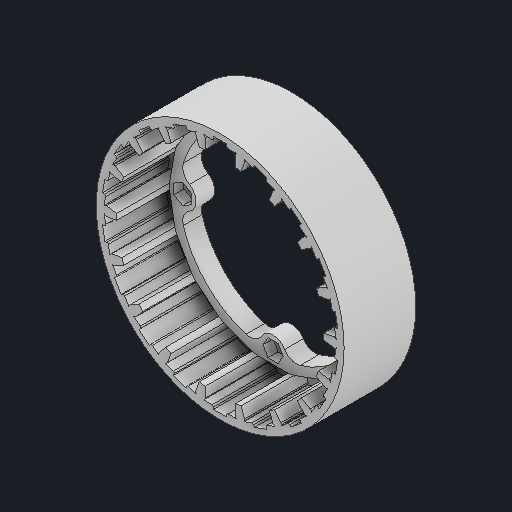
# Autodesk Inventor part: Rotator_A
Saved by Autodesk Inventor 2025.1 (Build 291241020, 241B)
## iProperties
Created: 2025-07-24
Part Number: Rotator_A
Material: 일반
Document SubType Name: Modeling
Designer: acalo
Density: 1 g/cm^3
Appearance: 기본값
Author: acalo
Autodesk Inventor part; units mm, degrees
ref_plane "YZ Plane" through (0, 0, 0) normal (1, 0, 0) x (0, 1, 0)
ref_plane "XZ Plane" through (0, 0, 0) normal (0, 1, 0) x (-1, 0, 0)
ref_plane "XY Plane" through (0, 0, 0) normal (0, 0, 1) x (1, 0, 0)
sketch "스케치1" plane through (0, 0, 0) normal (0, 0, 1) x (1, 0, 0)
  circle A0 centre (0, 0) radius 30
  line L0 (0, 30) -> (0, 30.6)
  line L1 (0, 30.6) -> (4.5, 30.6)
  line L2 (4.5, 30.6) -> (4.5, 34.2)
  line L3 (4.5, 34.2) -> (-4.5, 34.2)
  line L4 (-4.5, 34.2) -> (-4.5, 30.6)
  line L5 (-4.5, 30.6) -> (0, 30.6)
  line L6 (-10.4658, 28.7546) -> (-6.2372, 30.2937)
  line L7 (-6.2372, 30.2937) -> (-7.4685, 33.6766)
  line L8 (-7.4685, 33.6766) -> (-15.9257, 30.5984)
  line L9 (-15.9257, 30.5984) -> (-14.6944, 27.2155)
  line L10 (-14.6944, 27.2155) -> (-10.4658, 28.7546)
  line L11 (-19.6693, 23.441) -> (-16.2221, 26.3335)
  line L12 (-16.2221, 26.3335) -> (-18.5361, 29.0913)
  line L13 (-18.5361, 29.0913) -> (-25.4305, 23.3062)
  line L14 (-25.4305, 23.3062) -> (-23.1165, 20.5484)
  line L15 (-23.1165, 20.5484) -> (-19.6693, 23.441)
  line L16 (-26.5004, 15.3) -> (-24.2504, 19.1971)
  line L17 (-24.2504, 19.1971) -> (-27.3681, 20.9971)
  line L18 (-27.3681, 20.9971) -> (-31.8681, 13.2029)
  line L19 (-31.8681, 13.2029) -> (-28.7504, 11.4029)
  line L20 (-28.7504, 11.4029) -> (-26.5004, 15.3)
  line L21 (-30.1351, 5.3136) -> (-29.3537, 9.7453)
  line L22 (-29.3537, 9.7453) -> (-32.899, 10.3704)
  line L23 (-32.899, 10.3704) -> (-34.4618, 1.5071)
  line L24 (-34.4618, 1.5071) -> (-30.9165, 0.882)
  line L25 (-30.9165, 0.882) -> (-30.1351, 5.3136)
  line L26 (-30.1351, -5.3136) -> (-30.9165, -0.882)
  line L27 (-30.9165, -0.882) -> (-34.4618, -1.5071)
  line L28 (-34.4618, -1.5071) -> (-32.899, -10.3704)
  line L29 (-32.899, -10.3704) -> (-29.3537, -9.7453)
  line L30 (-29.3537, -9.7453) -> (-30.1351, -5.3136)
  line L31 (-26.5004, -15.3) -> (-28.7504, -11.4029)
  line L32 (-28.7504, -11.4029) -> (-31.8681, -13.2029)
  line L33 (-31.8681, -13.2029) -> (-27.3681, -20.9971)
  line L34 (-27.3681, -20.9971) -> (-24.2504, -19.1971)
  line L35 (-24.2504, -19.1971) -> (-26.5004, -15.3)
  line L36 (-19.6693, -23.441) -> (-23.1165, -20.5484)
  line L37 (-23.1165, -20.5484) -> (-25.4305, -23.3062)
  line L38 (-25.4305, -23.3062) -> (-18.5361, -29.0913)
  line L39 (-18.5361, -29.0913) -> (-16.2221, -26.3335)
  line L40 (-16.2221, -26.3335) -> (-19.6693, -23.441)
  line L41 (-10.4658, -28.7546) -> (-14.6944, -27.2155)
  line L42 (-14.6944, -27.2155) -> (-15.9257, -30.5984)
  line L43 (-15.9257, -30.5984) -> (-7.4685, -33.6766)
  line L44 (-7.4685, -33.6766) -> (-6.2372, -30.2937)
  line L45 (-6.2372, -30.2937) -> (-10.4658, -28.7546)
  line L46 (0, -30.6) -> (-4.5, -30.6)
  line L47 (-4.5, -30.6) -> (-4.5, -34.2)
  line L48 (-4.5, -34.2) -> (4.5, -34.2)
  line L49 (4.5, -34.2) -> (4.5, -30.6)
  line L50 (4.5, -30.6) -> (0, -30.6)
  line L51 (10.4658, -28.7546) -> (6.2372, -30.2937)
  line L52 (6.2372, -30.2937) -> (7.4685, -33.6766)
  line L53 (7.4685, -33.6766) -> (15.9257, -30.5984)
  line L54 (15.9257, -30.5984) -> (14.6944, -27.2155)
  line L55 (14.6944, -27.2155) -> (10.4658, -28.7546)
  line L56 (19.6693, -23.441) -> (16.2221, -26.3335)
  line L57 (16.2221, -26.3335) -> (18.5361, -29.0913)
  line L58 (18.5361, -29.0913) -> (25.4305, -23.3062)
  line L59 (25.4305, -23.3062) -> (23.1165, -20.5484)
  line L60 (23.1165, -20.5484) -> (19.6693, -23.441)
  line L61 (26.5004, -15.3) -> (24.2504, -19.1971)
  line L62 (24.2504, -19.1971) -> (27.3681, -20.9971)
  line L63 (27.3681, -20.9971) -> (31.8681, -13.2029)
  line L64 (31.8681, -13.2029) -> (28.7504, -11.4029)
  line L65 (28.7504, -11.4029) -> (26.5004, -15.3)
  line L66 (30.1351, -5.3136) -> (29.3537, -9.7453)
  line L67 (29.3537, -9.7453) -> (32.899, -10.3704)
  line L68 (32.899, -10.3704) -> (34.4618, -1.5071)
  line L69 (34.4618, -1.5071) -> (30.9165, -0.882)
  line L70 (30.9165, -0.882) -> (30.1351, -5.3136)
  line L71 (30.1351, 5.3136) -> (30.9165, 0.882)
  line L72 (30.9165, 0.882) -> (34.4618, 1.5071)
  line L73 (34.4618, 1.5071) -> (32.899, 10.3704)
  line L74 (32.899, 10.3704) -> (29.3537, 9.7453)
  line L75 (29.3537, 9.7453) -> (30.1351, 5.3136)
  line L76 (26.5004, 15.3) -> (28.7504, 11.4029)
  line L77 (28.7504, 11.4029) -> (31.8681, 13.2029)
  line L78 (31.8681, 13.2029) -> (27.3681, 20.9971)
  line L79 (27.3681, 20.9971) -> (24.2504, 19.1971)
  line L80 (24.2504, 19.1971) -> (26.5004, 15.3)
  line L81 (19.6693, 23.441) -> (23.1165, 20.5484)
  line L82 (23.1165, 20.5484) -> (25.4305, 23.3062)
  line L83 (25.4305, 23.3062) -> (18.5361, 29.0913)
  line L84 (18.5361, 29.0913) -> (16.2221, 26.3335)
  line L85 (16.2221, 26.3335) -> (19.6693, 23.441)
  line L86 (10.4658, 28.7546) -> (14.6944, 27.2155)
  line L87 (14.6944, 27.2155) -> (15.9257, 30.5984)
  line L88 (15.9257, 30.5984) -> (7.4685, 33.6766)
  line L89 (7.4685, 33.6766) -> (6.2372, 30.2937)
  line L90 (6.2372, 30.2937) -> (10.4658, 28.7546)
  circle A1 centre (0, 0) radius 28
  circle A2 centre (0, 0) radius 37
  line L91 (-4.5, 30.6) -> (-6.2372, 30.2937)
  line L92 (-14.6944, 27.2155) -> (-16.2221, 26.3335)
  line L93 (-23.1165, 20.5484) -> (-24.2504, 19.1971)
  line L94 (-28.7504, 11.4029) -> (-29.3537, 9.7453)
  line L95 (-30.9165, 0.882) -> (-30.9165, -0.882)
  line L96 (-29.3537, -9.7453) -> (-28.7504, -11.4029)
  line L97 (-24.2504, -19.1971) -> (-23.1165, -20.5484)
  line L98 (-16.2221, -26.3335) -> (-14.6944, -27.2155)
  line L99 (-6.2372, -30.2937) -> (-4.5, -30.6)
  line L100 (4.5, -30.6) -> (6.2372, -30.2937)
  line L101 (14.6944, -27.2155) -> (16.2221, -26.3335)
  line L102 (23.1165, -20.5484) -> (24.2504, -19.1971)
  line L103 (28.7504, -11.4029) -> (29.3537, -9.7453)
  line L104 (30.9165, -0.882) -> (30.9165, 0.882)
  line L105 (29.3537, 9.7453) -> (28.7504, 11.4029)
  line L106 (24.2504, 19.1971) -> (23.1165, 20.5484)
  line L107 (16.2221, 26.3335) -> (14.6944, 27.2155)
  line L108 (6.2372, 30.2937) -> (4.5, 30.6)
  dimension "d1" = 0.6
  dimension "d2" = 4.5
  dimension "d3" = 3.6
  dimension "d4" = 9
  dimension "d7" = 360
  dimension "d9" = 56
  dimension "d10" = 74
  dimension "d13" = 360
  constraints: 218 end point, 18 point on line, 4 perpendicular, 3 coincident, 2 centre point, 1 horizontal, 1 vertical, 1 vertical alignment, 238 other
  measures "d1" distance of L0.start L0.end
  measures "d2" distance of L0.end L1.end
  measures "d3" distance of L1.end L2.end
  measures "d4" distance of L2.end L3.end
  measures "d9" diameter of A1
  measures "d10" diameter of A2
extrude "돌출1" add sketch "스케치1" along normal blind 19 contours A2
extrude "돌출2" add sketch "스케치1" against normal blind 2.4 contours A0 | L5 L4 L3 L2 L1 | L1 L108 L90 L86 L107 L85 L81 L106 L80 L76 L105 L75 L71 L104 L70 L66 L103 L65 L61 L102 L60 L56 L101 L55 L51 L100 L50 L46 L99 L45 L41 L98 L40 L36 L97 L35 L31 L96 L30 L26 L95 L25 L21 L94 L20 L16 L93 L15 L11 L92 L10 L6 L91 L5 | L89 L88 L87 L86 L90 | L6 L10 L9 L8 L7 | L84 L83 L82 L81 L85 | L11 L15 L14 L13 L12 | L79 L78 L77 L76 L80 | L16 L20 L19 L18 L17 | L74 L73 L72 L71 L75 | L21 L25 L24 L23 L22 | L69 L68 L67 L66 L70 | L26 L30 L29 L28 L27 | L64 L63 L62 L61 L65 | L31 L35 L34 L33 L32 | L59 L58 L57 L56 L60 | L36 L40 L39 L38 L37 | L54 L53 L52 L51 L55 | L41 L45 L44 L43 L42 | L49 L48 L47 L46 L50 | A2
extrude "돌출3" add sketch "스케치1" along normal blind 2 contours A0 | L1 L108 L90 L86 L107 L85 L81 L106 L80 L76 L105 L75 L71 L104 L70 L66 L103 L65 L61 L102 L60 L56 L101 L55 L51 L100 L50 L46 L99 L45 L41 L98 L40 L36 L97 L35 L31 L96 L30 L26 L95 L25 L21 L94 L20 L16 L93 L15 L11 L92 L10 L6 L91 L5
sketch "스케치2" plane through (0, 0, 19) normal (0, 0, 1) x (1, 0, 0)
  circle A0 centre (0, 0) radius 37 projected
  line L0 (4.5, 30.6) -> (6.2372, 30.2937) projected
  line L1 (6.2372, 30.2937) -> (7.4685, 33.6766) projected
  line L2 (7.4685, 33.6766) -> (15.9257, 30.5984) projected
  line L3 (15.9257, 30.5984) -> (14.6944, 27.2155) projected
  line L4 (14.6944, 27.2155) -> (16.2221, 26.3335) projected
  line L5 (16.2221, 26.3335) -> (18.5361, 29.0913) projected
  line L6 (18.5361, 29.0913) -> (25.4305, 23.3062) projected
  line L7 (25.4305, 23.3062) -> (23.1165, 20.5484) projected
  line L8 (23.1165, 20.5484) -> (24.2504, 19.1971) projected
  line L9 (24.2504, 19.1971) -> (27.3681, 20.9971) projected
  line L10 (27.3681, 20.9971) -> (31.8681, 13.2029) projected
  line L11 (31.8681, 13.2029) -> (28.7504, 11.4029) projected
  line L12 (28.7504, 11.4029) -> (29.3537, 9.7453) projected
  line L13 (29.3537, 9.7453) -> (32.899, 10.3704) projected
  line L14 (32.899, 10.3704) -> (34.4618, 1.5071) projected
  line L15 (34.4618, 1.5071) -> (30.9165, 0.882) projected
  line L16 (30.9165, 0.882) -> (30.9165, -0.882) projected
  line L17 (30.9165, -0.882) -> (34.4618, -1.5071) projected
  line L18 (34.4618, -1.5071) -> (32.899, -10.3704) projected
  line L19 (32.899, -10.3704) -> (29.3537, -9.7453) projected
  line L20 (29.3537, -9.7453) -> (28.7504, -11.4029) projected
  line L21 (28.7504, -11.4029) -> (31.8681, -13.2029) projected
  line L22 (31.8681, -13.2029) -> (27.3681, -20.9971) projected
  line L23 (27.3681, -20.9971) -> (24.2504, -19.1971) projected
  line L24 (24.2504, -19.1971) -> (23.1165, -20.5484) projected
  line L25 (23.1165, -20.5484) -> (25.4305, -23.3062) projected
  line L26 (25.4305, -23.3062) -> (18.5361, -29.0913) projected
  line L27 (18.5361, -29.0913) -> (16.2221, -26.3335) projected
  line L28 (16.2221, -26.3335) -> (14.6944, -27.2155) projected
  line L29 (14.6944, -27.2155) -> (15.9257, -30.5984) projected
  line L30 (15.9257, -30.5984) -> (7.4685, -33.6766) projected
  line L31 (7.4685, -33.6766) -> (6.2372, -30.2937) projected
  line L32 (6.2372, -30.2937) -> (4.5, -30.6) projected
  line L33 (4.5, -30.6) -> (4.5, -34.2) projected
  line L34 (4.5, -34.2) -> (-4.5, -34.2) projected
  line L35 (-4.5, -34.2) -> (-4.5, -30.6) projected
  line L36 (-4.5, -30.6) -> (-6.2372, -30.2937) projected
  line L37 (-6.2372, -30.2937) -> (-7.4685, -33.6766) projected
  line L38 (-7.4685, -33.6766) -> (-15.9257, -30.5984) projected
  line L39 (-15.9257, -30.5984) -> (-14.6944, -27.2155) projected
  line L40 (-14.6944, -27.2155) -> (-16.2221, -26.3335) projected
  line L41 (-16.2221, -26.3335) -> (-18.5361, -29.0913) projected
  line L42 (-18.5361, -29.0913) -> (-25.4305, -23.3062) projected
  line L43 (-25.4305, -23.3062) -> (-23.1165, -20.5484) projected
  line L44 (-23.1165, -20.5484) -> (-24.2504, -19.1971) projected
  line L45 (-24.2504, -19.1971) -> (-27.3681, -20.9971) projected
  line L46 (-27.3681, -20.9971) -> (-31.8681, -13.2029) projected
  line L47 (-31.8681, -13.2029) -> (-28.7504, -11.4029) projected
  line L48 (-28.7504, -11.4029) -> (-29.3537, -9.7453) projected
  line L49 (-29.3537, -9.7453) -> (-32.899, -10.3704) projected
  line L50 (-32.899, -10.3704) -> (-34.4618, -1.5071) projected
  line L51 (-34.4618, -1.5071) -> (-30.9165, -0.882) projected
  line L52 (-30.9165, -0.882) -> (-30.9165, 0.882) projected
  line L53 (-30.9165, 0.882) -> (-34.4618, 1.5071) projected
  line L54 (-34.4618, 1.5071) -> (-32.899, 10.3704) projected
  line L55 (-32.899, 10.3704) -> (-29.3537, 9.7453) projected
  line L56 (-29.3537, 9.7453) -> (-28.7504, 11.4029) projected
  line L57 (-28.7504, 11.4029) -> (-31.8681, 13.2029) projected
  line L58 (-31.8681, 13.2029) -> (-27.3681, 20.9971) projected
  line L59 (-27.3681, 20.9971) -> (-24.2504, 19.1971) projected
  line L60 (-24.2504, 19.1971) -> (-23.1165, 20.5484) projected
  line L61 (-23.1165, 20.5484) -> (-25.4305, 23.3062) projected
  line L62 (-25.4305, 23.3062) -> (-18.5361, 29.0913) projected
  line L63 (-18.5361, 29.0913) -> (-16.2221, 26.3335) projected
  line L64 (-16.2221, 26.3335) -> (-14.6944, 27.2155) projected
  line L65 (-14.6944, 27.2155) -> (-15.9257, 30.5984) projected
  line L66 (-15.9257, 30.5984) -> (-7.4685, 33.6766) projected
  line L67 (-7.4685, 33.6766) -> (-6.2372, 30.2937) projected
  line L68 (-6.2372, 30.2937) -> (-4.5, 30.6) projected
  line L69 (-4.5, 30.6) -> (-4.5, 34.2) projected
  line L70 (-4.5, 34.2) -> (4.5, 34.2) projected
  line L71 (4.5, 34.2) -> (4.5, 30.6) projected
  line L72 (37, 0) -> (38.2, 0)
  circle A1 centre (38.2, 0) radius 1.65
  line L73 (38.2, 0) -> (42.2, 0)
  arc A2 (42.01, -4) -> (42.01, 4) centre (0, 0) ccw
  line L74 (36.7831, 4) -> (42.01, 4)
  line L75 (36.7831, -4) -> (42.01, -4)
  point P0 (38.2, 4)
  point P1 (40.3945, 4)
  point P2 (38.2, -4)
  point P3 (40.3945, -4)
  point P4 (36.9832, 1.1144)
  point P5 (36.9832, -1.1144)
  dimension "d22" = 3.3
  dimension "d27" = 4
  constraints: 8 end point, 6 point on circle, 4 point on line, 2 centre point, 2 coincident, 2 horizontal, 2 symmetric about line
  measures "d22" diameter of A1
  measures "d27" distance of L73.start L73.end
thicken "두껍게 하기1" operation add thickness 1.2 both sides no extend neighbours no toward (0, 0, 1) faces at (-1.125, 29.6653, 2)
sketch "스케치3" plane through (0, 0, 19) normal (0, 0, 1) x (1, 0, 0)
  line L0 (4.2, -34.2) -> (-4.2, -34.2)
  line L1 (4.5, -34.2) -> (-4.5, -34.2)
  line L2 (0, -35.2) -> (-2, -35.2)
  line L3 (-2, -35.2) -> (-2, -34.2)
  line L4 (0, -35.2) -> (2, -35.2)
  line L5 (2, -35.2) -> (2, -34.2)
  point P0 (0, 0)
  dimension "d40" = 2
  constraints: 12 end point, 2 point on line
  measures "d40" distance of L2.start L2.end
extrude "돌출6" cut sketch "스케치3" against normal up to surface (19 mm away)
fillet "모깎기3" radius 0.4 2 edges at (2, -34.2, 9.5) (-2, -34.2, 9.5)
pattern_circular "원형 패턴3" count 18 over 360 about axis through (0, 0, 0) along (0, 0, -1) of "모깎기3", "돌출6"
ref_plane "작업 평면1" through (-4.2, -30.6, 3.2) normal (0, 0, 1) x (1, 0, 0)
sketch "스케치4" plane through (-4.2, -30.6, 3.2) normal (0, 0, 1) x (1, 0, 0)
  circle A0 centre (4.2, 30.6) radius 28 projected
  circle A1 centre (31.2, 30.6) radius 1.65
  line L0 (31.2, 34.6) -> (33.9128, 34.6)
  line L1 (31.2, 26.6) -> (33.9128, 26.6)
  arc A2 (31.2, 34.6) -> (31.2, 26.6) centre (31.2, 30.6) ccw
  line L2 (9.911, 34.0794) -> (11.911, 34.0794)
  point P0 (30.85, 34.6)
  point P1 (30.85, 26.6)
  point P2 (31.9128, 34.6)
  point P3 (31.9128, 26.6)
  point P4 (32.1681, 29.2639)
  point P5 (32.1681, 31.9361)
  dimension "d49" = 3.3
  dimension "d59" = 2
  constraints: 6 end point, 2 centre point, 2 horizontal, 2 point on circle, 1 coincident, 1 tangent
  measures "d49" diameter of A1
  measures "d59" distance of L2.start L2.end
extrude "돌출10" add sketch "스케치4" against normal up to surface (5.6 mm away) contours A1 A0 L1 A2 L0
extrude "돌출11" cut sketch "스케치4" against normal up to surface (5.6 mm away) contours A0 A1 | L0 A2 L1 A0 picked at (32.4002, 30.3229)
ref_plane "작업 평면2" through (-4.2, -30.6, 3.2) normal (0, 0, 1) x (1, 0, 0)
sketch "스케치7" plane through (-4.2, -30.6, 3.2) normal (0, 0, 1) x (1, 0, 0)
  circle A0 centre (31.2, 30.6) radius 1.65
  arc A1 (31.0117, 38.6704) -> (31.0117, 22.5296) centre (4.2, 30.6) ccw
  arc A2 (29.1907, 34.0587) -> (31.0117, 38.6704) centre (27.1815, 37.5175) ccw
  arc A3 (29.1907, 34.0587) -> (29.1907, 27.1413) centre (31.2, 30.6) ccw
  arc A4 (31.0117, 22.5296) -> (29.1907, 27.1413) centre (27.1815, 23.6825) ccw
  line L0 (-2.0372, 60.8937) -> (-0.3, 61.2) projected
  line L1 (-2.1398, 61.1756) -> (-2.0372, 60.8937) projected
  arc A5 (-2.3191, 60.7911) -> (-2.1398, 61.1756) centre (-2.4217, 61.073) ccw projected
  line L2 (-2.3191, 60.7911) -> (-10.2125, 57.9181) projected
  arc A6 (-10.597, 58.0974) -> (-10.2125, 57.9181) centre (-10.3151, 58.2) ccw projected
  line L3 (-10.4944, 57.8155) -> (-10.597, 58.0974) projected
  line L4 (-12.0221, 56.9335) -> (-10.4944, 57.8155) projected
  line L5 (-12.2149, 57.1633) -> (-12.0221, 56.9335) projected
  arc A7 (-12.2519, 56.7407) -> (-12.2149, 57.1633) centre (-12.4448, 56.9705) ccw projected
  line L6 (-12.2519, 56.7407) -> (-18.6867, 51.3413) projected
  arc A8 (-19.1093, 51.3782) -> (-18.6867, 51.3413) centre (-18.8795, 51.5711) ccw projected
  line L7 (-18.9165, 51.1484) -> (-19.1093, 51.3782) projected
  line L8 (-20.0504, 49.7971) -> (-18.9165, 51.1484) projected
  line L9 (-20.3102, 49.9471) -> (-20.0504, 49.7971) projected
  arc A9 (-20.2004, 49.5373) -> (-20.3102, 49.9471) centre (-20.4602, 49.6873) ccw projected
  line L10 (-20.2004, 49.5373) -> (-24.4004, 42.2627) projected
  arc A10 (-24.8102, 42.1529) -> (-24.4004, 42.2627) centre (-24.6602, 42.4127) ccw projected
  line L11 (-24.5504, 42.0029) -> (-24.8102, 42.1529) projected
  line L12 (-25.1537, 40.3453) -> (-24.5504, 42.0029) projected
  line L13 (-25.4491, 40.3974) -> (-25.1537, 40.3453) projected
  arc A11 (-25.2058, 40.0498) -> (-25.4491, 40.3974) centre (-25.5012, 40.1019) ccw projected
  line L14 (-25.2058, 40.0498) -> (-26.6644, 31.7774) projected
  arc A12 (-27.012, 31.5341) -> (-26.6644, 31.7774) centre (-26.9599, 31.8295) ccw projected
  line L15 (-26.7165, 31.482) -> (-27.012, 31.5341) projected
  line L16 (-26.7165, 29.718) -> (-26.7165, 31.482) projected
  line L17 (-27.012, 29.6659) -> (-26.7165, 29.718) projected
  arc A13 (-26.6644, 29.4226) -> (-27.012, 29.6659) centre (-26.9599, 29.3705) ccw projected
  line L18 (-26.6644, 29.4226) -> (-25.2058, 21.1502) projected
  arc A14 (-25.4491, 20.8026) -> (-25.2058, 21.1502) centre (-25.5012, 21.0981) ccw projected
  line L19 (-25.1537, 20.8547) -> (-25.4491, 20.8026) projected
  line L20 (-24.5504, 19.1971) -> (-25.1537, 20.8547) projected
  line L21 (-24.8102, 19.0471) -> (-24.5504, 19.1971) projected
  arc A15 (-24.4004, 18.9373) -> (-24.8102, 19.0471) centre (-24.6602, 18.7873) ccw projected
  line L22 (-24.4004, 18.9373) -> (-20.2004, 11.6627) projected
  arc A16 (-20.3102, 11.2529) -> (-20.2004, 11.6627) centre (-20.4602, 11.5127) ccw projected
  line L23 (-20.0504, 11.4029) -> (-20.3102, 11.2529) projected
  line L24 (-18.9165, 10.0516) -> (-20.0504, 11.4029) projected
  line L25 (-19.1093, 9.8218) -> (-18.9165, 10.0516) projected
  arc A17 (-18.6867, 9.8587) -> (-19.1093, 9.8218) centre (-18.8795, 9.6289) ccw projected
  line L26 (-18.6867, 9.8587) -> (-12.2519, 4.4593) projected
  arc A18 (-12.2149, 4.0367) -> (-12.2519, 4.4593) centre (-12.4448, 4.2295) ccw projected
  line L27 (-12.0221, 4.2665) -> (-12.2149, 4.0367) projected
  line L28 (-10.4944, 3.3845) -> (-12.0221, 4.2665) projected
  line L29 (-10.597, 3.1026) -> (-10.4944, 3.3845) projected
  arc A19 (-10.2125, 3.2819) -> (-10.597, 3.1026) centre (-10.3151, 3) ccw projected
  line L30 (-10.2125, 3.2819) -> (-2.3191, 0.4089) projected
  arc A20 (-2.1398, 0.0244) -> (-2.3191, 0.4089) centre (-2.4217, 0.127) ccw projected
  line L31 (-2.0372, 0.3063) -> (-2.1398, 0.0244) projected
  line L32 (-0.3, 0) -> (-2.0372, 0.3063) projected
  line L33 (-0.3, -0.3) -> (-0.3, 0) projected
  arc A21 (0, 0) -> (-0.3, -0.3) centre (0, -0.3) ccw projected
  line L34 (0, 0) -> (8.4, 0) projected
  arc A22 (8.7, -0.3) -> (8.4, 0) centre (8.4, -0.3) ccw projected
  line L35 (8.7, 0) -> (8.7, -0.3) projected
  line L36 (10.4372, 0.3063) -> (8.7, 0) projected
  line L37 (10.5398, 0.0244) -> (10.4372, 0.3063) projected
  arc A23 (10.7191, 0.4089) -> (10.5398, 0.0244) centre (10.8217, 0.127) ccw projected
  line L38 (10.7191, 0.4089) -> (18.6125, 3.2819) projected
  arc A24 (18.997, 3.1026) -> (18.6125, 3.2819) centre (18.7151, 3) ccw projected
  line L39 (18.8944, 3.3845) -> (18.997, 3.1026) projected
  line L40 (20.4221, 4.2665) -> (18.8944, 3.3845) projected
  line L41 (20.6149, 4.0367) -> (20.4221, 4.2665) projected
  arc A25 (20.6519, 4.4593) -> (20.6149, 4.0367) centre (20.8448, 4.2295) ccw projected
  line L42 (20.6519, 4.4593) -> (27.0867, 9.8587) projected
  arc A26 (27.5093, 9.8218) -> (27.0867, 9.8587) centre (27.2795, 9.6289) ccw projected
  line L43 (27.3165, 10.0516) -> (27.5093, 9.8218) projected
  line L44 (28.4504, 11.4029) -> (27.3165, 10.0516) projected
  line L45 (28.7102, 11.2529) -> (28.4504, 11.4029) projected
  arc A27 (28.6004, 11.6627) -> (28.7102, 11.2529) centre (28.8602, 11.5127) ccw projected
  line L46 (28.6004, 11.6627) -> (32.8004, 18.9373)
  arc A28 (33.2102, 19.0471) -> (32.8004, 18.9373) centre (33.0602, 18.7873) ccw
  line L47 (32.9504, 19.1971) -> (33.2102, 19.0471)
  line L48 (33.5537, 20.8547) -> (32.9504, 19.1971)
  line L49 (33.8491, 20.8026) -> (33.5537, 20.8547)
  arc A29 (33.6058, 21.1502) -> (33.8491, 20.8026) centre (33.9012, 21.0981) ccw
  line L50 (33.6058, 21.1502) -> (35.0644, 29.4226)
  arc A30 (35.412, 29.6659) -> (35.0644, 29.4226) centre (35.3599, 29.3705) ccw
  line L51 (35.1165, 29.718) -> (35.412, 29.6659)
  line L52 (35.1165, 31.482) -> (35.1165, 29.718)
  line L53 (35.412, 31.5341) -> (35.1165, 31.482)
  arc A31 (35.0644, 31.7774) -> (35.412, 31.5341) centre (35.3599, 31.8295) ccw
  line L54 (35.0644, 31.7774) -> (33.6058, 40.0498)
  arc A32 (33.8491, 40.3974) -> (33.6058, 40.0498) centre (33.9012, 40.1019) ccw
  line L55 (33.5537, 40.3453) -> (33.8491, 40.3974)
  line L56 (32.9504, 42.0029) -> (33.5537, 40.3453)
  line L57 (33.2102, 42.1529) -> (32.9504, 42.0029)
  arc A33 (32.8004, 42.2627) -> (33.2102, 42.1529) centre (33.0602, 42.4127) ccw
  line L58 (32.8004, 42.2627) -> (28.6004, 49.5373)
  arc A34 (28.7102, 49.9471) -> (28.6004, 49.5373) centre (28.8602, 49.6873) ccw projected
  line L59 (28.4504, 49.7971) -> (28.7102, 49.9471) projected
  line L60 (27.3165, 51.1484) -> (28.4504, 49.7971) projected
  line L61 (27.5093, 51.3782) -> (27.3165, 51.1484) projected
  arc A35 (27.0867, 51.3413) -> (27.5093, 51.3782) centre (27.2795, 51.5711) ccw projected
  line L62 (27.0867, 51.3413) -> (20.6519, 56.7407) projected
  arc A36 (20.6149, 57.1633) -> (20.6519, 56.7407) centre (20.8448, 56.9705) ccw projected
  line L63 (20.4221, 56.9335) -> (20.6149, 57.1633) projected
  line L64 (18.8944, 57.8155) -> (20.4221, 56.9335) projected
  line L65 (18.997, 58.0974) -> (18.8944, 57.8155) projected
  arc A37 (18.6125, 57.9181) -> (18.997, 58.0974) centre (18.7151, 58.2) ccw projected
  line L66 (18.6125, 57.9181) -> (10.7191, 60.7911) projected
  arc A38 (10.5398, 61.1756) -> (10.7191, 60.7911) centre (10.8217, 61.073) ccw projected
  line L67 (10.4372, 60.8937) -> (10.5398, 61.1756) projected
  line L68 (8.7, 61.2) -> (10.4372, 60.8937) projected
  line L69 (8.7, 61.5) -> (8.7, 61.2) projected
  arc A39 (8.4, 61.2) -> (8.7, 61.5) centre (8.4, 61.5) ccw projected
  line L70 (8.4, 61.2) -> (0, 61.2) projected
  arc A40 (-0.3, 61.5) -> (0, 61.2) centre (0, 61.5) ccw projected
  line L71 (-0.3, 61.2) -> (-0.3, 61.5) projected
  arc A41 (12.2704, 57.4117) -> (7.6587, 55.5907) centre (11.1175, 53.5815) ccw
  circle A42 centre (4.2, 57.6) radius 1.65
  arc A43 (0.7413, 55.5907) -> (7.6587, 55.5907) centre (4.2, 57.6) ccw
  arc A44 (0.7413, 55.5907) -> (-3.8704, 57.4117) centre (-2.7175, 53.5815) ccw
  arc A45 (-22.6117, 38.6704) -> (-20.7907, 34.0587) centre (-18.7815, 37.5175) ccw
  circle A46 centre (-22.8, 30.6) radius 1.65
  arc A47 (-20.7907, 27.1413) -> (-20.7907, 34.0587) centre (-22.8, 30.6) ccw
  arc A48 (-20.7907, 27.1413) -> (-22.6117, 22.5296) centre (-18.7815, 23.6825) ccw
  arc A49 (-3.8704, 3.7883) -> (0.7413, 5.6093) centre (-2.7175, 7.6185) ccw
  circle A50 centre (4.2, 3.6) radius 1.65
  arc A51 (7.6587, 5.6093) -> (0.7413, 5.6093) centre (4.2, 3.6) ccw
  arc A52 (7.6587, 5.6093) -> (12.2704, 3.7883) centre (11.1175, 7.6185) ccw
  point P0 (-23.7681, 31.9361)
  point P1 (-23.7681, 29.2639)
  point P2 (-3.8704, 3.7883)
  point P3 (2.8639, 2.6319)
  point P4 (5.5361, 2.6319)
  point P5 (12.2704, 3.7883)
  point P6 (12.2704, 57.4117)
  point P7 (5.5361, 58.5681)
  point P8 (2.8639, 58.5681)
  point P9 (-3.8704, 57.4117)
  dimension "d70" = 360
  constraints: 75 centre point, 38 point on circle, 26 end point, 49 other
extrude "돌출12" add sketch "스케치7" against normal up to surface (5.6 mm away) contours A41 A43 A44 A1 A42 | A1 A50 A49 A51 A52 | A45 A47 A48 A1 A46 | L0 L71 A40 L70 A39 L69 L68 L67 A38 L66 A37 L65 L64 L63 A36 L62 A35 L61 L60 L59 A34 L58 A33 L57 L56 L55 A32 L54 A31 L53 L52 L51 A30 L50 A29 L49 L48 L47 A28 L46 A27 L45 L44 L43 A26 L42 A25 L41 L40 L39 A24 L38 A23 L37 L36 L35 A22 L34 A21 L33 L32 L31 A20 L30 A19 L29 L28 L27 A18 L26 A17 L25 L24 L23 A16 L22 A15 L21 L20 L19 A14 L18 A13 L17 L16 L15 A12 L14 A11 L13 L12 L11 A10 L10 A9 L9 L8 L7 A8 L6 A7 L5 L4 L3 A6 L2 A5 L1
extrude "돌출13" cut sketch "스케치7" against normal blind 6 contours A42 A1 | A1 A42 | A50 A1 | A1 A50 | A46 A1 | A1 A46
ref_plane "작업 평면3" through (-4.2, -30.6, 3.2) normal (0, 0, 1) x (1, 0, 0)
sketch "스케치8" plane through (-4.2, -30.6, 3.2) normal (0, 0, 1) x (1, 0, 0)
  circle A0 centre (4.2, 57.6) radius 1.65 projected
  line L0 (4.2, 57.6) -> (4.2, 55)
  line L1 (2.6989, 55) -> (1.1978, 57.6)
  line L2 (1.1978, 57.6) -> (2.6989, 60.2)
  line L3 (2.6989, 60.2) -> (5.7011, 60.2)
  line L4 (5.7011, 60.2) -> (7.2022, 57.6)
  line L5 (7.2022, 57.6) -> (5.7011, 55)
  line L6 (5.7011, 55) -> (2.6989, 55)
  point P0 (4.2, 30.6)
  dimension "d76" = 2.6
  constraints: 14 end point, 1 coincident, 1 midpoint, 1 vertical, 13 other
  measures "d76" distance of L0.start L0.end
extrude "돌출14" cut sketch "스케치8" against normal blind 3
sketch "스케치9" plane through (0, 0, 19) normal (0, 0, 1) x (1, 0, 0)
  arc A0 (9.9545, -33.1974) -> (9.4418, -32.9583) centre (9.5786, -33.3342) ccw projected
  line L0 (9.4418, -32.9583) -> (7.4685, -33.6766) projected
  line L1 (7.4685, -33.6766) -> (6.2372, -30.2937) projected
  line L2 (6.2372, -30.2937) -> (4.5, -30.6) projected
  line L3 (4.5, -30.6) -> (4.5, -34.2) projected
  line L4 (4.5, -34.2) -> (2.4, -34.2) projected
  arc A1 (2.4, -34.2) -> (2, -34.6) centre (2.4, -34.6) ccw projected
  line L5 (2, -34.6) -> (2, -35.2) projected
  line L6 (2, -35.2) -> (-2, -35.2) projected
  line L7 (-2, -35.2) -> (-2, -34.6) projected
  arc A2 (-2, -34.6) -> (-2.4, -34.2) centre (-2.4, -34.6) ccw projected
  line L8 (-2.4, -34.2) -> (-4.5, -34.2) projected
  line L9 (-4.5, -34.2) -> (-4.5, -30.6) projected
  line L10 (-4.5, -30.6) -> (-6.2372, -30.2937) projected
  line L11 (-6.2372, -30.2937) -> (-7.4685, -33.6766) projected
  line L12 (-7.4685, -33.6766) -> (-9.4418, -32.9583) projected
  arc A3 (-9.4418, -32.9583) -> (-9.9545, -33.1974) centre (-9.5786, -33.3342) ccw projected
  line L13 (-9.9545, -33.1974) -> (-10.1597, -33.7612) projected
  line L14 (-10.1597, -33.7612) -> (-13.9185, -32.3931) projected
  line L15 (-13.9185, -32.3931) -> (-13.7133, -31.8293) projected
  arc A4 (-13.7133, -31.8293) -> (-13.9524, -31.3166) centre (-14.0892, -31.6925) ccw projected
  line L16 (-13.9524, -31.3166) -> (-15.9257, -30.5984) projected
  line L17 (-15.9257, -30.5984) -> (-14.6944, -27.2155) projected
  line L18 (-14.6944, -27.2155) -> (-16.2221, -26.3335) projected
  line L19 (-16.2221, -26.3335) -> (-18.5361, -29.0913) projected
  line L20 (-18.5361, -29.0913) -> (-20.1448, -27.7414) projected
  arc A5 (-20.1448, -27.7414) -> (-20.7084, -27.7907) centre (-20.4019, -28.0478) ccw projected
  line L21 (-20.7084, -27.7907) -> (-21.094, -28.2503) projected
  line L22 (-21.094, -28.2503) -> (-24.1582, -25.6792) projected
  line L23 (-24.1582, -25.6792) -> (-23.7725, -25.2196) projected
  arc A6 (-23.7725, -25.2196) -> (-23.8218, -24.656) centre (-24.079, -24.9624) ccw projected
  line L24 (-23.8218, -24.656) -> (-25.4305, -23.3062) projected
  line L25 (-25.4305, -23.3062) -> (-23.1165, -20.5484) projected
  line L26 (-23.1165, -20.5484) -> (-24.2504, -19.1971) projected
  line L27 (-24.2504, -19.1971) -> (-27.3681, -20.9971) projected
  line L28 (-27.3681, -20.9971) -> (-28.4181, -19.1785) projected
  arc A7 (-28.4181, -19.1785) -> (-28.9645, -19.0321) centre (-28.7645, -19.3785) ccw projected
  line L29 (-28.9645, -19.0321) -> (-29.4841, -19.3321) projected
  line L30 (-29.4841, -19.3321) -> (-31.4841, -15.8679) projected
  line L31 (-31.4841, -15.8679) -> (-30.9645, -15.5679) projected
  arc A8 (-30.9645, -15.5679) -> (-30.8181, -15.0215) centre (-31.1645, -15.2215) ccw projected
  line L32 (-30.8181, -15.0215) -> (-31.8681, -13.2029) projected
  line L33 (-31.8681, -13.2029) -> (-28.7504, -11.4029) projected
  line L34 (-28.7504, -11.4029) -> (-29.3537, -9.7453) projected
  line L35 (-29.3537, -9.7453) -> (-32.899, -10.3704) projected
  line L36 (-32.899, -10.3704) -> (-33.2637, -8.3023) projected
  arc A9 (-33.2637, -8.3023) -> (-33.7271, -7.9778) centre (-33.6576, -8.3718) ccw projected
  line L37 (-33.7271, -7.9778) -> (-34.3179, -8.082) projected
  line L38 (-34.3179, -8.082) -> (-35.0125, -4.1428) projected
  line L39 (-35.0125, -4.1428) -> (-34.4216, -4.0386) projected
  arc A10 (-34.4216, -4.0386) -> (-34.0972, -3.5752) centre (-34.4911, -3.6447) ccw projected
  line L40 (-34.0972, -3.5752) -> (-34.4618, -1.5071) projected
  line L41 (-34.4618, -1.5071) -> (-30.9165, -0.882) projected
  line L42 (-30.9165, -0.882) -> (-30.9165, 0.882) projected
  line L43 (-30.9165, 0.882) -> (-34.4618, 1.5071) projected
  line L44 (-34.4618, 1.5071) -> (-34.0972, 3.5752) projected
  arc A11 (-34.0972, 3.5752) -> (-34.4216, 4.0386) centre (-34.4911, 3.6447) ccw projected
  line L45 (-34.4216, 4.0386) -> (-35.0125, 4.1428) projected
  line L46 (-35.0125, 4.1428) -> (-34.3179, 8.082) projected
  line L47 (-34.3179, 8.082) -> (-33.7271, 7.9778) projected
  arc A12 (-33.7271, 7.9778) -> (-33.2637, 8.3023) centre (-33.6576, 8.3718) ccw projected
  line L48 (-33.2637, 8.3023) -> (-32.899, 10.3704) projected
  line L49 (-32.899, 10.3704) -> (-29.3537, 9.7453) projected
  line L50 (-29.3537, 9.7453) -> (-28.7504, 11.4029) projected
  line L51 (-28.7504, 11.4029) -> (-31.8681, 13.2029) projected
  line L52 (-31.8681, 13.2029) -> (-30.8181, 15.0215) projected
  arc A13 (-30.8181, 15.0215) -> (-30.9645, 15.5679) centre (-31.1645, 15.2215) ccw projected
  line L53 (-30.9645, 15.5679) -> (-31.4841, 15.8679) projected
  line L54 (-31.4841, 15.8679) -> (-29.4841, 19.3321) projected
  line L55 (-29.4841, 19.3321) -> (-28.9645, 19.0321) projected
  arc A14 (-28.9645, 19.0321) -> (-28.4181, 19.1785) centre (-28.7645, 19.3785) ccw projected
  line L56 (-28.4181, 19.1785) -> (-27.3681, 20.9971) projected
  line L57 (-27.3681, 20.9971) -> (-24.2504, 19.1971) projected
  line L58 (-24.2504, 19.1971) -> (-23.1165, 20.5484) projected
  line L59 (-23.1165, 20.5484) -> (-25.4305, 23.3062) projected
  line L60 (-25.4305, 23.3062) -> (-23.8218, 24.656) projected
  arc A15 (-23.8218, 24.656) -> (-23.7725, 25.2196) centre (-24.079, 24.9624) ccw projected
  line L61 (-23.7725, 25.2196) -> (-24.1582, 25.6792) projected
  line L62 (-24.1582, 25.6792) -> (-21.094, 28.2503) projected
  line L63 (-21.094, 28.2503) -> (-20.7084, 27.7907) projected
  arc A16 (-20.7084, 27.7907) -> (-20.1448, 27.7414) centre (-20.4019, 28.0478) ccw projected
  line L64 (-20.1448, 27.7414) -> (-18.5361, 29.0913) projected
  line L65 (-18.5361, 29.0913) -> (-16.2221, 26.3335) projected
  line L66 (-16.2221, 26.3335) -> (-14.6944, 27.2155) projected
  line L67 (-14.6944, 27.2155) -> (-15.9257, 30.5984) projected
  line L68 (-15.9257, 30.5984) -> (-13.9524, 31.3166) projected
  arc A17 (-13.9524, 31.3166) -> (-13.7133, 31.8293) centre (-14.0892, 31.6925) ccw projected
  line L69 (-13.7133, 31.8293) -> (-13.9185, 32.3931) projected
  line L70 (-13.9185, 32.3931) -> (-10.1597, 33.7612) projected
  line L71 (-10.1597, 33.7612) -> (-9.9545, 33.1974) projected
  arc A18 (-9.9545, 33.1974) -> (-9.4418, 32.9583) centre (-9.5786, 33.3342) ccw projected
  line L72 (-9.4418, 32.9583) -> (-7.4685, 33.6766) projected
  line L73 (-7.4685, 33.6766) -> (-6.2372, 30.2937) projected
  line L74 (-6.2372, 30.2937) -> (-4.5, 30.6)
  line L75 (-4.5, 30.7) -> (-4.5, 34.3)
  line L76 (-4.5, 34.3) -> (-2.4, 34.3)
  arc A19 (-2.4, 34.3) -> (-2, 34.7) centre (-2.4, 34.7) ccw
  line L77 (-2, 34.7) -> (-2, 35.3)
  line L78 (-2, 35.3) -> (2, 35.3)
  line L79 (2, 35.3) -> (2, 34.7)
  arc A20 (2, 34.7) -> (2.4, 34.3) centre (2.4, 34.7) ccw
  line L80 (2.4, 34.3) -> (4.5, 34.3)
  line L81 (4.5, 34.3) -> (4.5, 30.7)
  line L82 (4.5, 30.6) -> (6.2372, 30.2937)
  line L83 (6.2372, 30.2937) -> (7.4685, 33.6766) projected
  line L84 (7.4685, 33.6766) -> (9.4418, 32.9583) projected
  arc A21 (9.4418, 32.9583) -> (9.9545, 33.1974) centre (9.5786, 33.3342) ccw projected
  line L85 (9.9545, 33.1974) -> (10.1597, 33.7612) projected
  line L86 (10.1597, 33.7612) -> (13.9185, 32.3931) projected
  line L87 (13.9185, 32.3931) -> (13.7133, 31.8293) projected
  arc A22 (13.7133, 31.8293) -> (13.9524, 31.3166) centre (14.0892, 31.6925) ccw projected
  line L88 (13.9524, 31.3166) -> (15.9257, 30.5984) projected
  line L89 (15.9257, 30.5984) -> (14.6944, 27.2155) projected
  line L90 (14.6944, 27.2155) -> (16.2221, 26.3335) projected
  line L91 (16.2221, 26.3335) -> (18.5361, 29.0913) projected
  line L92 (18.5361, 29.0913) -> (20.1448, 27.7414) projected
  arc A23 (20.1448, 27.7414) -> (20.7084, 27.7907) centre (20.4019, 28.0478) ccw projected
  line L93 (20.7084, 27.7907) -> (21.094, 28.2503) projected
  line L94 (21.094, 28.2503) -> (24.1582, 25.6792) projected
  line L95 (24.1582, 25.6792) -> (23.7725, 25.2196) projected
  arc A24 (23.7725, 25.2196) -> (23.8218, 24.656) centre (24.079, 24.9624) ccw projected
  line L96 (23.8218, 24.656) -> (25.4305, 23.3062) projected
  line L97 (25.4305, 23.3062) -> (23.1165, 20.5484) projected
  line L98 (23.1165, 20.5484) -> (24.2504, 19.1971) projected
  line L99 (24.2504, 19.1971) -> (27.3681, 20.9971) projected
  line L100 (27.3681, 20.9971) -> (28.4181, 19.1785) projected
  arc A25 (28.4181, 19.1785) -> (28.9645, 19.0321) centre (28.7645, 19.3785) ccw projected
  line L101 (28.9645, 19.0321) -> (29.4841, 19.3321) projected
  line L102 (29.4841, 19.3321) -> (31.4841, 15.8679) projected
  line L103 (31.4841, 15.8679) -> (30.9645, 15.5679) projected
  arc A26 (30.9645, 15.5679) -> (30.8181, 15.0215) centre (31.1645, 15.2215) ccw projected
  line L104 (30.8181, 15.0215) -> (31.8681, 13.2029) projected
  line L105 (31.8681, 13.2029) -> (28.7504, 11.4029) projected
  line L106 (28.7504, 11.4029) -> (29.3537, 9.7453) projected
  line L107 (29.3537, 9.7453) -> (32.899, 10.3704) projected
  line L108 (32.899, 10.3704) -> (33.2637, 8.3023) projected
  arc A27 (33.2637, 8.3023) -> (33.7271, 7.9778) centre (33.6576, 8.3718) ccw projected
  line L109 (33.7271, 7.9778) -> (34.3179, 8.082) projected
  line L110 (34.3179, 8.082) -> (35.0125, 4.1428) projected
  line L111 (35.0125, 4.1428) -> (34.4216, 4.0386) projected
  arc A28 (34.4216, 4.0386) -> (34.0972, 3.5752) centre (34.4911, 3.6447) ccw projected
  line L112 (34.0972, 3.5752) -> (34.4618, 1.5071) projected
  line L113 (34.4618, 1.5071) -> (30.9165, 0.882) projected
  line L114 (30.9165, 0.882) -> (30.9165, -0.882) projected
  line L115 (30.9165, -0.882) -> (34.4618, -1.5071) projected
  line L116 (34.4618, -1.5071) -> (34.0972, -3.5752) projected
  arc A29 (34.0972, -3.5752) -> (34.4216, -4.0386) centre (34.4911, -3.6447) ccw projected
  line L117 (34.4216, -4.0386) -> (35.0125, -4.1428) projected
  line L118 (35.0125, -4.1428) -> (34.3179, -8.082) projected
  line L119 (34.3179, -8.082) -> (33.7271, -7.9778) projected
  arc A30 (33.7271, -7.9778) -> (33.2637, -8.3023) centre (33.6576, -8.3718) ccw projected
  line L120 (33.2637, -8.3023) -> (32.899, -10.3704) projected
  line L121 (32.899, -10.3704) -> (29.3537, -9.7453) projected
  line L122 (29.3537, -9.7453) -> (28.7504, -11.4029) projected
  line L123 (28.7504, -11.4029) -> (31.8681, -13.2029) projected
  line L124 (31.8681, -13.2029) -> (30.8181, -15.0215) projected
  arc A31 (30.8181, -15.0215) -> (30.9645, -15.5679) centre (31.1645, -15.2215) ccw projected
  line L125 (30.9645, -15.5679) -> (31.4841, -15.8679) projected
  line L126 (31.4841, -15.8679) -> (29.4841, -19.3321) projected
  line L127 (29.4841, -19.3321) -> (28.9645, -19.0321) projected
  arc A32 (28.9645, -19.0321) -> (28.4181, -19.1785) centre (28.7645, -19.3785) ccw projected
  line L128 (28.4181, -19.1785) -> (27.3681, -20.9971) projected
  line L129 (27.3681, -20.9971) -> (24.2504, -19.1971) projected
  line L130 (24.2504, -19.1971) -> (23.1165, -20.5484) projected
  line L131 (23.1165, -20.5484) -> (25.4305, -23.3062) projected
  line L132 (25.4305, -23.3062) -> (23.8218, -24.656) projected
  arc A33 (23.8218, -24.656) -> (23.7725, -25.2196) centre (24.079, -24.9624) ccw projected
  line L133 (23.7725, -25.2196) -> (24.1582, -25.6792) projected
  line L134 (24.1582, -25.6792) -> (21.094, -28.2503) projected
  line L135 (21.094, -28.2503) -> (20.7084, -27.7907) projected
  arc A34 (20.7084, -27.7907) -> (20.1448, -27.7414) centre (20.4019, -28.0478) ccw projected
  line L136 (20.1448, -27.7414) -> (18.5361, -29.0913) projected
  line L137 (18.5361, -29.0913) -> (16.2221, -26.3335) projected
  line L138 (16.2221, -26.3335) -> (14.6944, -27.2155) projected
  line L139 (14.6944, -27.2155) -> (15.9257, -30.5984) projected
  line L140 (15.9257, -30.5984) -> (13.9524, -31.3166) projected
  arc A35 (13.9524, -31.3166) -> (13.7133, -31.8293) centre (14.0892, -31.6925) ccw projected
  line L141 (13.7133, -31.8293) -> (13.9185, -32.3931) projected
  line L142 (13.9185, -32.3931) -> (10.1597, -33.7612) projected
  line L143 (10.1597, -33.7612) -> (9.9545, -33.1974) projected
  circle A36 centre (0, 0) radius 37 projected
  circle A37 centre (0, 0) radius 30
  line L144 (0.226, 31.8293) -> (0.226, 31.9293)
  line L145 (-4.5, 34.2) -> (-2.4, 34.2) projected
  arc A38 (-2.4, 34.2) -> (-2, 34.6) centre (-2.4, 34.6) ccw projected
  line L146 (-2, 34.6) -> (-2, 35.2) projected
  line L147 (2, 35.2) -> (2, 34.6) projected
  line L148 (-4.2, 30.6) -> (4.2, 30.6) projected
  line L149 (4.5, 34.2) -> (4.5, 30.9) projected
  line L150 (2.4, 34.2) -> (4.5, 34.2) projected
  arc A39 (2, 34.6) -> (2.4, 34.2) centre (2.4, 34.6) ccw projected
  line L151 (2, 35.2) -> (2, 34.6) projected
  line L152 (-2, 35.2) -> (2, 35.2) projected
  line L153 (-2, 34.6) -> (-2, 35.2) projected
  arc A40 (-2.4, 34.2) -> (-2, 34.6) centre (-2.4, 34.6) ccw projected
  line L154 (-4.5, 34.2) -> (-2.4, 34.2) projected
  line L155 (-4.5, 30.9) -> (-4.5, 34.2) projected
  line L156 (2.4, 34.2) -> (4.5, 34.2) projected
  line L157 (-4.5, 34.3) -> (-4.9, 34.3)
  line L158 (-4.9, 34.3) -> (-4.5, 33.9)
  line L159 (0, 35.3) -> (0, 36.2338)
  line L160 (4.5, 34.3) -> (4.9, 34.3)
  line L161 (4.9, 34.3) -> (4.5, 33.9)
  arc A41 (-4.5, 30.9) -> (-4.2, 30.6) centre (-4.2, 30.9) ccw projected
  arc A42 (4.2, 30.6) -> (4.5, 30.9) centre (4.2, 30.9) ccw projected
  point P0 (4.5, 33.9)
  point P1 (-4.5, 33.9)
  dimension "d82" = 60
  dimension "d83" = 0.1
  dimension "d84" = 0.4
  dimension "d85" = 45
  constraints: 40 centre point, 30 end point, 4 point on circle, 4 vertical, 2 symmetric about line, 1 coincident, 1 horizontal, 1 midpoint, 1 point on line
  measures "d82" diameter of A37
  measures "d83" distance of L144.start L144.end
  measures "d84" distance of L75.end L157.end
  measures "d85" angle of L158 L157
extrude "돌출15" cut sketch "스케치9" against normal up to surface (19 mm away) contours L158 L157 L75 | L75 L76 A19 L146 A38 L145 | L81 L160 L161 | L150 A39 L147 A20 L80 L81 | L77 L78 L79 L152
fillet "모깎기7" radius 0.6 2 edges at (-4.5, 33.9, 9.5) (4.5, 33.9, 9.5)
pattern_circular "원형 패턴6" count 18 over 360 about axis through (0, 0, 0) along (0, 0, -1) of "돌출15", "모깎기7"
pattern_circular "원형 패턴7" count 4 over 360 about axis through (0, 0, 0) along (0, 0, -1) of "돌출14"
